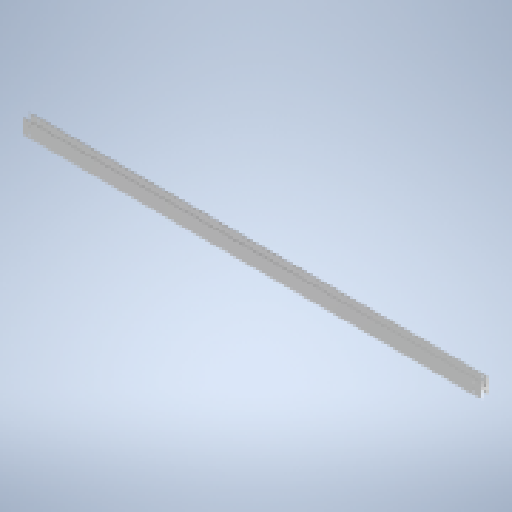
# Autodesk Inventor part: Träger
Saved by Autodesk Inventor 2025 (Build 290162010, 162A)
## iProperties
Created: 2024-11-07
Part Number: Träger
Material: Aluminium 6061, Träger
Document SubType Name: Modeling
Designer: Admin
Density: 2.7 g/cm^3
Appearance: Aluminium - flach(1)
Mass: 340.2 g
Surface Area: 1602.52 cm^2
Volume: 126 cm^3
Author: Admin
Autodesk Inventor part; units mm, degrees
ref_plane "YZ Plane" through (0, 0, 0) normal (1, 0, 0) x (0, 1, 0)
ref_plane "XZ Plane" through (0, 0, 0) normal (0, 1, 0) x (-1, 0, 0)
ref_plane "XY Plane" through (0, 0, 0) normal (0, 0, 1) x (1, 0, 0)
sketch "Skizze1" plane through (0, 0, 0) normal (1, 0, 0) x (0, 1, 0)
  line L0 (9, 16) -> (9, -16)
  line L1 (9, -16) -> (7.5, -16)
  line L2 (7.5, -16) -> (7.5, -1)
  line L3 (7.5, -1) -> (-7.5, -1)
  line L4 (-7.5, -1) -> (-7.5, -16)
  line L5 (-7.5, -16) -> (-9, -16)
  line L6 (-9, -16) -> (-9, 16)
  line L7 (-9, 16) -> (-7.5, 16)
  line L8 (-7.5, 16) -> (-7.5, 1)
  line L9 (-7.5, 1) -> (7.5, 1)
  line L10 (9, 16) -> (7.5, 16)
  line L11 (7.5, 16) -> (7.5, 1)
  line L12 (0, 0) -> (9, 0) construction
  line L13 (0, 0) -> (-9, 0) construction
  line L14 (0, 0) -> (0, 16) construction
  line L15 (0, 0) -> (0, -16) construction
  dimension "d0" = 2
  dimension "d1" = 1.5
  dimension "d2" = 32
  dimension "d3" = 18
  constraints: 32 end point, 11 perpendicular, 8 equal length, 5 point on line, 2 midpoint, 1 coincident, 1 horizontal, 1 vertical
  measures "d0" distance between parallel lines of L3 L9
  measures "d1" distance between parallel lines of L11 L0
  measures "d2" distance of L0.start L0.end
  measures "d3" distance of L5.end L0.end
extrude "Extrusion1" add sketch "Skizze1" along normal mid plane 1000
sketch "Skizze2" plane through (-500, 9, 16) normal (0, 1, 0) x (1, 0, 0)
  line L0 (985, 23.5) -> (985, 8.5)
  line L1 (15, 23.5) -> (15, 8.5)
  line L2 (15, 16) -> (0, 16)
  line L3 (0, 0) -> (0, 32) projected
  line L4 (1000, 32) -> (1000, 0) projected
  line L5 (985, 16) -> (1000, 16)
  point P0 (500, 16)
  dimension "d6" = 15
  dimension "d8" = 15
  dimension "d9" = 15
  dimension "d17" = 8.5
  dimension "d18" = 15
  constraints: 8 end point, 4 midpoint, 2 perpendicular, 2 vertical
  measures "d6" distance of L0.start L0.end
  measures "d8" distance of L1.start L1.end
  measures "d9" distance of L2.start L2.end
  measures "d17" vertical distance of L3.start L1.end
  measures "d18" distance of L5.start L5.end
hole "Bohrung1" at (485, 9, -7.5) at (485, 9, 7.5) at (-485, 9, -7.5) at (-485, 9, 7.5) direction (0, -1, 0) diameter 5 end through all
